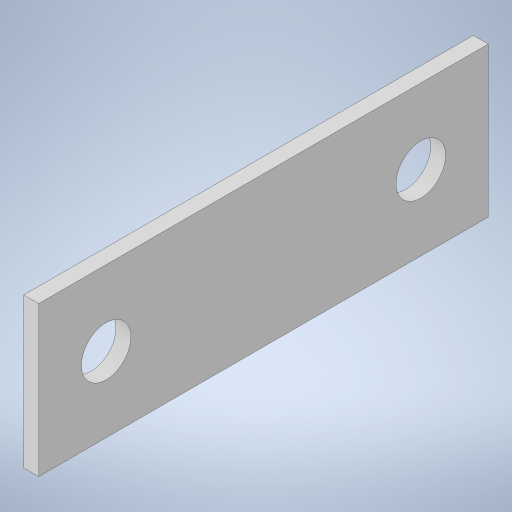
# Autodesk Inventor part: encorder_spacer
Saved by Autodesk Inventor 2024 (Build 280153000, 153)
## iProperties
Created: 2025-07-03
Part Number: encorder_spacer
Material: 一般
Document SubType Name: Modeling
Designer: HosodaLab2
Density: 1 g/cm^3
Appearance: 既定
Author: HosodaLab2
Autodesk Inventor part; units mm, degrees
ref_plane "YZ Plane" through (0, 0, 0) normal (1, 0, 0) x (0, 1, 0)
ref_plane "XZ Plane" through (0, 0, 0) normal (0, 1, 0) x (-1, 0, 0)
ref_plane "XY Plane" through (0, 0, 0) normal (0, 0, 1) x (1, 0, 0)
sketch "スケッチ1" plane through (0, 0, 0) normal (0, 1, 0) x (-1, 0, 0)
  line L0 (0, 0) -> (-30, 0)
  line L1 (-30, 0) -> (-30, -10)
  line L2 (-30, -10) -> (0, -10)
  line L3 (0, -10) -> (0, 0)
  dimension "d0" = 30
  dimension "d1" = 10
  constraints: 8 end point, 2 parallel, 1 horizontal, 1 perpendicular
  measures "d0" distance of L2.end L1.end
  measures "d1" distance of L1.end L0.end
extrude "押し出し1" add sketch "スケッチ1" along normal blind 1
sketch "スケッチ2" plane through (0, 1, 0) normal (0, 1, 0) x (1, 0, 0)
  line L0 (0, 10) -> (0, 0) construction
  line L1 (0, 5) -> (30, 5) construction
  line L2 (30, 0) -> (30, 10) construction
  point P0 (4.5, 5)
  point P1 (25.5, 5)
  dimension "d4" = 21
  dimension "d5" = 4.5
  constraints: 2 end point, 2 midpoint, 2 point on line
  measures "d4" distance of point (25.5, 5) point (4.5, 5)
  measures "d5" distance from line of point (4.5, 5) L0
hole "穴1" at (4.5, 1, -5) at (25.5, 1, -5) direction (0, -1, 0) diameter 3.3 depth 2 tip angle 118
